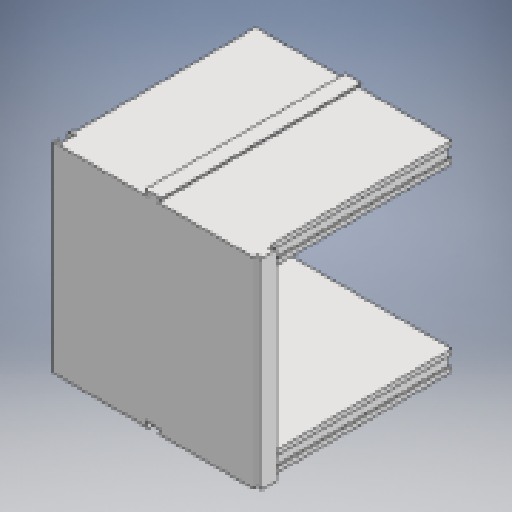
# Autodesk Inventor part: mainframe
Saved by Autodesk Inventor 2025.2 (Build 292293000, 293)
## iProperties
Created: 2025-02-22
Part Number: mainframe
Material: Generic
Document SubType Name: Modeling
Designer: email
Density: 1 g/cm^3
Appearance: Default
Author: email
Autodesk Inventor part; units mm, degrees
ref_plane "YZ Plane" through (0, 0, 0) normal (1, 0, 0) x (0, 1, 0)
ref_plane "XZ Plane" through (0, 0, 0) normal (0, 1, 0) x (-1, 0, 0)
ref_plane "XY Plane" through (0, 0, 0) normal (0, 0, 1) x (1, 0, 0)
sketch "Sketch1" plane through (0, 0, 0) normal (1, 0, 0) x (0, 1, 0)
  line L0 (0, 0) -> (100, 0)
  line L1 (100, 0) -> (100, -100)
  line L2 (100, -100) -> (90, -100)
  line L3 (90, -100) -> (90, -10)
  line L4 (90, -10) -> (10, -10)
  line L5 (10, -10) -> (10, -100)
  line L6 (10, -100) -> (0, -100)
  line L7 (0, -100) -> (0, 0)
  dimension "d0" = 100
  dimension "d1" = 100
  dimension "d2" = 10
  dimension "d3" = 10
  dimension "d4" = 10
  constraints: 16 end point, 6 perpendicular, 2 point on line, 1 horizontal
  measures "d0" distance of L0.end L1.end
  measures "d1" distance between parallel lines of L7 L1
  measures "d2" distance between parallel lines of L1 L3
  measures "d3" distance between parallel lines of L7 L5
  measures "d4" distance between parallel lines of L0 L4
extrude "Extrusion1" add sketch "Sketch1" against normal blind 100
sketch "Sketch2" plane through (0, 90, -100) normal (0, 0, -1) x (-1, 0, 0)
  line L0 (50, -90) -> (50, 10) construction
  line L1 (0, -40) -> (100, -40) construction
  line L2 (100, 0) -> (100, -80) projected
  line L3 (0, -90) -> (100, -90) projected
  line L4 (0, 10) -> (100, 10) projected
  line L5 (1, 10) -> (1, 7.5)
  line L6 (1, 7.5) -> (3.5, 9)
  line L7 (3.5, 9) -> (3.5, 1)
  line L8 (3.5, 1) -> (1, 2.5)
  line L9 (1, 2.5) -> (1, -40)
  line L10 (0, 0) -> (0, 10) projected
  line L11 (99, 10) -> (99, 7.5)
  line L12 (99, 7.5) -> (96.5, 9)
  line L13 (96.5, 9) -> (96.5, 1)
  line L14 (96.5, 1) -> (99, 2.5)
  line L15 (99, 2.5) -> (99, -40)
  line L16 (100, 0) -> (100, 10)
  line L17 (0, -90) -> (100, -90)
  line L18 (1, -90) -> (1, -87.5)
  line L19 (1, -87.5) -> (3.5, -89)
  line L20 (3.5, -89) -> (3.5, -81)
  line L21 (3.5, -81) -> (1, -82.5)
  line L22 (1, -82.5) -> (1, -40)
  line L23 (0, -80) -> (0, -90)
  line L24 (99, -82.5) -> (99, -40)
  line L25 (96.5, -81) -> (99, -82.5)
  line L26 (96.5, -89) -> (96.5, -81)
  line L27 (99, -87.5) -> (96.5, -89)
  line L28 (100, -80) -> (100, -90)
  line L29 (99, -90) -> (99, -87.5)
  line L30 (0, 10) -> (100, 10)
  line L31 (100, 10) -> (100, -90)
  line L32 (100, -90) -> (0, -90)
  line L33 (0, -90) -> (0, 10)
  point P0 (50, -40)
  dimension "d12" = 2.5
  dimension "d14" = 8
  dimension "d15" = 2.5
  dimension "d16" = 1
  dimension "d18" = 1
  dimension "d19" = 59.036
  constraints: 60 end point, 17 symmetric about line, 4 midpoint, 3 point on line, 3 vertical, 2 parallel, 2 perpendicular, 1 collinear, 1 horizontal
  measures "d12" distance of L5.start L5.end
  measures "d14" distance of L6.end L7.end
  measures "d15" distance between parallel lines of L5 L7
  measures "d16" distance between parallel lines of L10 L5
  measures "d18" distance from line of L4 L6.end
  measures "d19" angle of L8 L7
extrude "Extrusion2" cut sketch "Sketch2" against normal blind 90 contours L2 L28 L3 L29 L27 L26 L25 L24 L15 L14 L13 L12 L11 L4 L16 | L5 L6 L7 L8 L9 L22 L21 L20 L19 L18 L3 L23 L33 L10 L4
sketch "Sketch3" plane through (0, 100, 0) normal (0, 1, 0) x (1, 0, 0)
  line L0 (0, 0) -> (0, 10) projected
  line L1 (0, 0) -> (0, 2.5)
  line L2 (0, 2.5) -> (2.5, 1)
  line L3 (2.5, 1) -> (2.5, 9)
  line L4 (2.5, 9) -> (0, 7.5)
  line L5 (0, 10) -> (0, 0) projected
  line L6 (-1, 10) -> (0, 10) projected
  line L7 (0, 10) -> (0, 7.5)
  line L8 (0, 0) -> (-100, 0) projected
  line L9 (-97.5, 1) -> (-97.5, 9)
  line L10 (-97.5, 9) -> (-100, 7.5)
  line L11 (-100, 0) -> (-100, 10) projected
  line L12 (-100, 7.5) -> (-100, 2.5)
  line L13 (-97.5, 1) -> (-100, 2.5)
  dimension "d22" = 2.5
  dimension "d23" = 2.5
  dimension "d24" = 8
  dimension "d25" = 2.5
  dimension "d26" = 1
  dimension "d27" = 2.5
  dimension "d28" = 2.5
  dimension "d29" = 8
  dimension "d30" = 2.5
  dimension "d31" = 1
  constraints: 18 end point, 4 point on line, 2 vertical, 1 parallel
  measures "d22" distance of L1.end L0.start
  measures "d23" distance of L0.end L4.end
  measures "d24" distance of L2.end L3.end
  measures "d25" distance between parallel lines of L0 L3
  measures "d26" distance from line of L8 L2.end
  measures "d27" distance from line of L8 L12.end
  measures "d28" distance of L11.end L10.end
  measures "d29" distance of L9.start L9.end
  measures "d30" distance between parallel lines of L11 L9
  measures "d31" distance from line of L8 L9.start
extrude "Extrusion3" add sketch "Sketch3" against normal up to surface (100 mm away) contours L0 L4 L3 L2
extrude "Extrusion4" cut sketch "Sketch3" against normal up to surface (100 mm away) contours L13 L11 L10 L9
sketch "Sketch4" plane through (-1, 90, -100) normal (0, 0, -1) x (-1, 0, 0)
  line L0 (0, -90) -> (98, -90) projected
  line L1 (46.5, -90) -> (45, -87.5)
  line L2 (45, -87.5) -> (53, -87.5)
  line L3 (53, -87.5) -> (51.5, -90)
  line L4 (0, 10) -> (98, 10) projected
  line L5 (49, 10) -> (49, -90) construction
  line L6 (46.5, -90) -> (51.5, -90)
  line L7 (45, 12.5) -> (53, 12.5)
  line L8 (53, 12.5) -> (51.5, 10)
  line L9 (42.8887, 10) -> (51.5, 10)
  line L10 (45, 12.5) -> (46.5, 10)
  line L11 (51.5, 10) -> (46.5, 10)
  point P0 (-1, -90)
  point P1 (49, -87.5)
  point P2 (49, -40)
  point P3 (49, -90)
  point P4 (49, 12.5)
  dimension "d36" = 8
  dimension "d37" = 2.5
  dimension "d38" = 5
  dimension "d39" = 2.5
  dimension "d40" = 8
  dimension "d42" = 5
  constraints: 20 end point, 9 midpoint, 4 point on line, 3 collinear, 3 vertical alignment, 1 coincident, 1 parallel
  measures "d36" distance of L1.end L2.end
  measures "d37" distance between parallel lines of L0 L2
  measures "d38" distance of L3.end L1.start
  measures "d39" distance between parallel lines of L4 L7
  measures "d40" distance of L7.start L7.end
  measures "d42" distance of L8.end L10.end
extrude "Extrusion5" add sketch "Sketch4" against normal up to surface (100 mm away) contours L10 L7 L8 L4
extrude "Extrusion6" cut sketch "Sketch4" against normal up to surface (100 mm away) contours L1 L2 L3 L0
sketch "Sketch7" plane through (-1, 90, -100) normal (1, 0, 0) x (0, 0, -1)
  line L0 (0, 10) -> (0, 7.5) projected
  line L1 (-90, -87.5) -> (-90, -90) projected
  line L2 (0, 10) -> (-90, 10)
  line L3 (-90, 10) -> (-90, -90)
  line L4 (-90, -90) -> (0, -90)
  line L5 (0, -90) -> (0, 10)
  point P0 (-100, -90)
  constraints: 8 end point, 2 parallel, 1 horizontal, 1 perpendicular
extrude "Extrusion9" cut sketch "Sketch7" against normal blind 0.1
sketch "Sketch8" plane through (-96.5, 91, -100) normal (0, 0, -1) x (-1, 0, 0)
  line L0 (-96.5, 9) -> (-49, 9) projected
  line L1 (-42.5, 11.5) -> (-50.5, 11.5) projected
  line L2 (-49, 9) -> (-50.5, 11.5)
  line L3 (-50.5, 11.5) -> (-42.5, 11.5)
  line L4 (-44, 9) -> (-42.5, 11.5) projected
  line L5 (-42.5, 11.5) -> (-44, 9)
  line L6 (-49, 9) -> (-44, 9)
  line L7 (-42.6766, 11.4) -> (-44.1166, 9)
  line L8 (-50.3234, 11.4) -> (-48.8834, 9)
  line L9 (-50.3234, 11.4) -> (-42.6766, 11.4)
  point P0 (-96.5, -91)
  dimension "d59" = 0.1
  dimension "d60" = 0.1
  dimension "d61" = 0.1
  constraints: 14 end point, 2 collinear, 2 point on line, 1 horizontal
  measures "d59" distance between parallel lines of L4 L7
  measures "d60" distance between parallel lines of L1 L9
  measures "d61" distance between parallel lines of L2 L8
extrude "Extrusion10" cut sketch "Sketch8" against normal up to surface (100 mm away) contours L4 L6 L7 L9 L8 L2 L1
sketch "Sketch9" plane through (-99, 97.5, -100) normal (-1, 0, 0) x (0, 0, 1)
  line L0 (0, 2.5) -> (90, 2.5) projected
  line L1 (90, 2.5) -> (90, -97.5) projected
  line L2 (0, 2.5) -> (90, 2.5)
  line L3 (90, 2.5) -> (90, -97.5)
  line L4 (90, -97.5) -> (0, -97.5)
  line L5 (0, -97.5) -> (0, 2.5)
  point P0 (100, -97.5)
  constraints: 8 end point, 2 parallel, 1 horizontal, 1 perpendicular
extrude "Extrusion11" cut sketch "Sketch9" against normal blind 0.1
sketch "Sketch10" plane through (2.5, 100, -1) normal (0, 1, 0) x (1, 0, 0)
  line L0 (0, 8) -> (-2.5, 6.5) projected
  line L1 (-2.5, 6.5) -> (0, 8)
  line L2 (-2.5, 1.5) -> (0, 0) projected
  line L3 (0, 8) -> (0, 0)
  line L4 (0, 0) -> (-2.5, 1.5)
  line L5 (-2.5, 6.3834) -> (-0.1, 7.8234)
  line L6 (-0.1, 7.8234) -> (-0.1, 0.1766)
  line L7 (-0.1, 0.1766) -> (-2.5, 1.6166)
  line L8 (0, 8) -> (-2.5, 6.5) projected
  line L9 (-2.5, 6.5) -> (-2.5, 9) projected
  line L10 (-2.5, 6.5) -> (-2.5, 1.5)
  point P0 (-2.5, -1)
  dimension "d66" = 0.1
  dimension "d67" = 0.1
  dimension "d68" = 0.1
  constraints: 14 end point, 3 collinear, 3 parallel, 2 point on line, 1 vertical
  measures "d66" distance between parallel lines of L0 L5
  measures "d67" distance between parallel lines of L2 L7
  measures "d68" distance between parallel lines of L3 L6
extrude "Extrusion12" cut sketch "Sketch10" against normal through all contours L3 L2 L10 L7 L6 L5 L0
body "Solid1"
